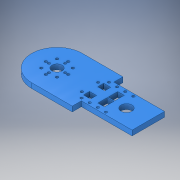
# Autodesk Inventor part: 000.401 - Опорная платформа
Saved by Autodesk Inventor 2019 (Build 230136000, 136)
## iProperties
Created: 2020-03-18
Part Number: 000.401 - Опорная платформа
Material: Пластик АБС
Document SubType Name: Modeling
Designer: Петров Иван
Density: 1.06 g/cm^3
Appearance: Голубой
Author: Петров Иван
Autodesk Inventor part; units mm, degrees
ref_plane "YZ Plane" through (0, 0, 0) normal (1, 0, 0) x (0, 1, 0)
ref_plane "XZ Plane" through (0, 0, 0) normal (0, 1, 0) x (-1, 0, 0)
ref_plane "XY Plane" through (0, 0, 0) normal (0, 0, 1) x (1, 0, 0)
sketch "Эскиз1" plane through (0, 0, 0) normal (0, 1, 0) x (-1, 0, 0)
  circle A0 centre (0, 0) radius 13.8
  circle A1 centre (-8, 0) radius 1.2
  circle A2 centre (0, -8) radius 1.2
  circle A3 centre (8, 0) radius 1.2
  circle A4 centre (0, 8) radius 1.2
  circle A5 centre (-7.7782, 7.7782) radius 1.2813
  circle A6 centre (-11, 0) radius 1.2813
  circle A7 centre (-7.7782, -7.7782) radius 1.2813
  circle A8 centre (0, -11) radius 1.2812
  circle A9 centre (7.7782, -7.7782) radius 1.2812
  circle A10 centre (11, 0) radius 1.2813
  circle A11 centre (7.7782, 7.7782) radius 1.2812
  circle A12 centre (0, 11) radius 1.2812
  circle A13 centre (0, 0) radius 5
  circle A14 centre (0, 0) radius 14
  circle A15 centre (0, 0) radius 1.55
  circle A16 centre (0, 0) radius 1.75
  circle A17 centre (0, 0) radius 25
  dimension "d0" = 50
  constraints: 18 centre point, 1 coincident
  measures "d0" diameter of A17
extrude "Выдавливание1" add sketch "Эскиз1" along normal blind 5 contours A0 | A14 | A17
sketch "Эскиз2" plane through (0, 5, 0) normal (0, 1, 0) x (1, 0, 0)
  line L0 (25, 0) -> (100, 0)
  circle A0 centre (100, 0) radius 25
  line L1 (50, 0) -> (50, -20)
  line L2 (50, 0) -> (50, 20)
  circle A1 centre (0, 0) radius 25 projected
  arc A2 (4.9455, 24.506) -> (95.0545, 24.506) centre (50, 247.5) ccw
  arc A3 (95.0545, -24.506) -> (4.9455, -24.506) centre (50, -247.5) ccw
  line L3 (100, 25) -> (0, 25)
  line L4 (0, -25) -> (100, -25)
  line L5 (50, 20) -> (50, 25)
  line L6 (50, -20) -> (50, -25)
  line L7 (50, 25) -> (50, -25)
  dimension "d3" = 100
  dimension "d4" = 50
  dimension "d5" = 20
  dimension "d6" = 20
  constraints: 16 end point, 15 point on circle, 3 centre point, 3 tangent, 2 midpoint, 2 vertical, 1 coincident, 1 collinear, 1 horizontal, 1 point on line
  measures "d3" distance of point (0, 0) L0.end
  measures "d4" diameter of A0
  measures "d5" distance of L1.start L1.end
  measures "d6" distance of L1.start L2.end
extrude "Выдавливание2" add sketch "Эскиз2" against normal blind 5 contours A1 A2 L2 L0 | L0 L1 A3 A1 | A1 L3 L5 A2 | A3 L6 L4 A1
sketch "Эскиз7" plane through (0, 5, 0) normal (0, 1, 0) x (1, 0, 0)
  line L0 (100, 0) -> (100, 15)
  line L1 (100, 0) -> (100, -15)
  circle A0 centre (100, 15) radius 3
  circle A1 centre (100, -15) radius 3
  line L2 (100, 0) -> (115, 0)
  circle A2 centre (115, 0) radius 3
  point P0 (0, 0)
  dimension "d23" = 15
  dimension "d24" = 15
  dimension "d25" = 6
  dimension "d26" = 6
  dimension "d27" = 15
  dimension "d28" = 6
  constraints: 6 end point, 3 centre point, 3 coincident, 2 vertical, 1 horizontal, 1 other
  measures "d23" distance of L0.start L0.end
  measures "d24" distance of L0.start L1.end
  measures "d25" diameter of A0
  measures "d26" diameter of A1
  measures "d27" distance of L0.start L2.end
  measures "d28" diameter of A2
extrude "Выдавливание7" [suppressed]
move faces "Перенос1" translate (40, 0, 0) faces at (50, 3.3333, 8.3333)
sketch "Эскиз10" plane through (0, 5, 0) normal (0, 1, 0) x (1, 0, 0)
  line L0 (65, -15) -> (65, -13)
  line L1 (65, -13) -> (66.5, -13)
  line L2 (66.5, -13) -> (66.5, -12)
  line L3 (66.5, -12) -> (75, -12)
  arc A0 (75, -12) -> (79, -8) centre (75, -8) ccw
  line L4 (79, -8) -> (79, 8)
  arc A1 (79, 8) -> (75, 12) centre (75, 8) ccw
  line L5 (75, 12) -> (66.5, 12)
  line L6 (66.5, 12) -> (66.5, 13)
  line L7 (66.5, 13) -> (65, 13)
  line L8 (65, 13) -> (65, 15)
  line L9 (65, 15) -> (58.5, 15)
  line L10 (58.5, 15) -> (58.5, 13)
  line L11 (58.5, 13) -> (57, 13)
  line L12 (57, 13) -> (57, 15)
  line L13 (57, 15) -> (50.5, 15)
  line L14 (50.5, 15) -> (50.5, 13)
  line L15 (50.5, 13) -> (49, 13)
  line L16 (49, 13) -> (49, 15)
  line L17 (49, 15) -> (42.5, 15)
  line L18 (42.5, 15) -> (42.5, 13)
  line L19 (42.5, 13) -> (41, 13)
  line L20 (41, 13) -> (41, 15)
  line L21 (41, 15) -> (34.5, 15)
  line L22 (34.5, 15) -> (34.5, 13)
  line L23 (34.5, 13) -> (33, 13)
  line L24 (33, 13) -> (33, 11.25)
  line L25 (33, 11.25) -> (31, 11.25)
  line L26 (31, 11.25) -> (31, 4.75)
  line L27 (31, 4.75) -> (33, 4.75)
  line L28 (33, 4.75) -> (33, -4.75)
  line L29 (33, -4.75) -> (31, -4.75)
  line L30 (31, -4.75) -> (31, -11.25)
  line L31 (31, -11.25) -> (33, -11.25)
  line L32 (33, -11.25) -> (33, -13)
  line L33 (33, -13) -> (34.5, -13)
  line L34 (34.5, -13) -> (34.5, -15)
  line L35 (34.5, -15) -> (41, -15)
  line L36 (41, -15) -> (41, -13)
  line L37 (41, -13) -> (42.5, -13)
  line L38 (42.5, -13) -> (42.5, -15)
  line L39 (42.5, -15) -> (49, -15)
  line L40 (49, -15) -> (49, -13)
  line L41 (49, -13) -> (50.5, -13)
  line L42 (50.5, -13) -> (50.5, -15)
  line L43 (50.5, -15) -> (57, -15)
  line L44 (57, -15) -> (57, -13)
  line L45 (57, -13) -> (58.5, -13)
  line L46 (58.5, -13) -> (58.5, -15)
  line L47 (58.5, -15) -> (65, -15)
  line L48 (36, -4.3) -> (36, -9.7)
  arc A2 (36.3, -4) -> (36, -4.3) centre (36.3, -4.3) ccw
  line L49 (42.7, -4) -> (36.3, -4)
  arc A3 (43, -4.3) -> (42.7, -4) centre (42.7, -4.3) ccw
  line L50 (43, -9.7) -> (43, -4.3)
  arc A4 (42.7, -10) -> (43, -9.7) centre (42.7, -9.7) ccw
  line L51 (36.3, -10) -> (42.7, -10)
  arc A5 (36, -9.7) -> (36.3, -10) centre (36.3, -9.7) ccw
  circle A6 centre (32.5, -8) radius 1.25
  circle A7 centre (37.75, -13.5) radius 1.25
  circle A8 centre (45.75, -13.5) radius 1.25
  circle A9 centre (53.75, -13.5) radius 1.25
  circle A10 centre (61.75, -13.5) radius 1.25
  circle A11 centre (32.5, 8) radius 1.25
  circle A12 centre (45.75, 13.5) radius 1.25
  circle A13 centre (61.75, 13.5) radius 1.25
  circle A14 centre (76, 6) radius 1
  circle A15 centre (62.5, -8) radius 1
  circle A16 centre (47, -8) radius 1
  circle A17 centre (76, -6) radius 1
  circle A18 centre (47, 8) radius 1
  circle A19 centre (62.5, 8) radius 1
  circle A20 centre (68.5, 0) radius 5.4
  line L52 (50, 0.5) -> (50, 9.8)
  line L53 (50, 9.8) -> (56.5, 9.8)
  line L54 (56.5, 9.8) -> (56.5, 0.5)
  line L55 (50, 0.5) -> (56.5, 0.5)
  line L56 (56.5, -0.5) -> (56.5, -9.8)
  line L57 (56.5, -9.8) -> (50, -9.8)
  line L58 (50, -9.8) -> (50, -0.5)
  line L59 (56.5, -0.5) -> (50, -0.5)
  circle A21 centre (53.75, 13.5) radius 1.25
  circle A22 centre (37.75, 13.5) radius 1.25
  line L60 (42.7, 10) -> (36.3, 10)
  arc A23 (43, 9.7) -> (42.7, 10) centre (42.7, 9.7) ccw
  line L61 (43, 4.3) -> (43, 9.7)
  arc A24 (42.7, 4) -> (43, 4.3) centre (42.7, 4.3) ccw
  line L62 (36.3, 4) -> (42.7, 4)
  arc A25 (36, 4.3) -> (36.3, 4) centre (36.3, 4.3) ccw
  line L63 (36, 9.7) -> (36, 4.3)
  arc A26 (36.3, 10) -> (36, 9.7) centre (36.3, 9.7) ccw
  line L64 (75, -13) -> (66.5, -13)
  arc A27 (75, -13) -> (80, -8) centre (75, -8) ccw
  line L65 (80, 8) -> (80, -8)
  arc A28 (80, 8) -> (75, 13) centre (75, 8) ccw
  line L66 (66.5, 13) -> (75, 13)
  line L67 (66.5, 14.5) -> (66.5, 13)
  line L68 (65, 14.5) -> (66.5, 14.5)
  line L69 (58.5, 16) -> (65, 16)
  line L70 (65, 16) -> (65, 15)
  line L71 (58.5, 15) -> (58.5, 16)
  line L72 (50.5, 16) -> (57, 16)
  line L73 (57, 16) -> (57, 15)
  line L74 (50.5, 15) -> (50.5, 16)
  line L75 (49, 16) -> (49, 15)
  line L76 (42.5, 15) -> (42.5, 16)
  line L77 (42.5, 16) -> (49, 16)
  line L78 (34.5, 16) -> (41, 16)
  line L79 (41, 16) -> (41, 15)
  line L80 (34.5, 15) -> (34.5, 16)
  line L81 (33, 14.5) -> (34.5, 14.5)
  line L82 (34.5, 14.5) -> (34.5, 13)
  line L83 (33, 14.5) -> (34.5, 14.5)
  line L84 (33, 13) -> (33, 14.5)
  line L85 (34.5, 13) -> (33, 13)
  line L86 (31.5, 13) -> (33, 13)
  line L87 (31.5, 13) -> (33, 13)
  line L88 (31.5, 11.25) -> (31.5, 13)
  line L89 (33, 11.25) -> (31.5, 11.25)
  line L90 (33, 13) -> (33, 11.25)
  line L91 (30, 4.75) -> (30, 11.25)
  line L92 (30, 11.25) -> (31, 11.25)
  line L93 (30, 4.75) -> (30, 11.25)
  line L94 (31, 4.75) -> (30, 4.75)
  line L95 (31, 11.25) -> (31, 4.75)
  line L96 (30, -4.75) -> (31, -4.75)
  line L97 (30, -11.25) -> (30, -4.75)
  line L98 (31, -11.25) -> (30, -11.25)
  line L99 (31, -4.75) -> (31, -11.25)
  line L100 (31.5, -11.25) -> (33, -11.25)
  line L101 (31.5, -13) -> (31.5, -11.25)
  line L102 (33, -13) -> (31.5, -13)
  line L103 (33, -11.25) -> (33, -13)
  line L104 (33, -14.5) -> (33, -13)
  line L105 (34.5, -14.5) -> (33, -14.5)
  line L106 (34.5, -13) -> (34.5, -14.5)
  line L107 (33, -13) -> (34.5, -13)
  line L108 (34.5, -16) -> (34.5, -15)
  line L109 (41, -16) -> (34.5, -16)
  line L110 (41, -15) -> (41, -16)
  line L111 (34.5, -15) -> (41, -15)
  line L112 (42.5, -16) -> (42.5, -15)
  line L113 (49, -16) -> (42.5, -16)
  line L114 (49, -15) -> (49, -16)
  line L115 (42.5, -15) -> (49, -15)
  line L116 (50.5, -16) -> (50.5, -15)
  line L117 (57, -16) -> (50.5, -16)
  line L118 (57, -15) -> (57, -16)
  line L119 (50.5, -15) -> (57, -15)
  line L120 (58.5, -16) -> (58.5, -15)
  line L121 (65, -16) -> (58.5, -16)
  line L122 (65, -15) -> (65, -16)
  line L123 (58.5, -15) -> (65, -15)
  line L124 (65, -14.5) -> (65, -13)
  line L125 (66.5, -14.5) -> (65, -14.5)
  line L126 (66.5, -13) -> (66.5, -14.5)
  line L127 (65, -13) -> (66.5, -13)
  line L128 (90, -25) -> (90, 25) projected
  point P0 (0, 0)
  point P1 (68.5, 0)
  point P2 (80, 0)
  point P3 (90, 0)
  constraints: 256 end point, 29 centre point, 24 point on circle, 2 midpoint
extrude "Выдавливание10" cut sketch "Эскиз10" against normal blind 10 contours A2 L49 A3 L50 A4 L51 A5 L48 | A6 | A7 | A8 | A9 | A10 | A11 | A12 | A13 | A20 | L52 L53 L54 L55 | L56 L57 L58 L59 | A21 | A22 | A23 L61 A24 L62 A25 L63 A26 L60
sketch "Эскиз11" plane through (0, 5, 0) normal (0, 1, 0) x (1, 0, 0)
  line L0 (90, -25) -> (0, -25) projected
  line L1 (90, -25) -> (40, -25)
  line L2 (40, -25) -> (40, -16)
  line L3 (40, -16) -> (90, -16)
  line L4 (90, -16) -> (90, -25)
  point P0 (0, 0)
  dimension "d41" = 50
  dimension "d42" = 9
  constraints: 8 end point, 2 parallel, 1 horizontal, 1 perpendicular
  measures "d41" distance of L2.end L3.end
  measures "d42" distance of L1.end L2.end
extrude "Выдавливание11" cut sketch "Эскиз11" against normal blind 10
mirror "Зеркальное отражение2" about plane through (0, 0, 0) normal (0, 0, 1) of "Выдавливание11"
equation "\"d6\" = d5"
equation "\"d24\" = d23"
equation "\"d26\" = d25"
equation "\"d27\" = d23"
equation "\"d28\" = d25"
